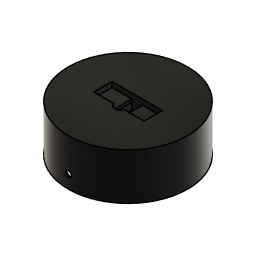
Base V2 - USB C v6 (Autodesk Fusion 360 design; units mm, degrees)
Autodesk Fusion 360 part; units mm, degrees
note: some values were not read from the file. Set by a fixed rule: which face or edge a step refers to.
sketch "Schizzo1" plane through (0, 0, 0) normal (0, 1, 0) x (1, 0, 0)
  circle A0 centre (0, 0) radius 45
  dimension "d1" = 90
  constraint coincident A0.centre origin
  measures "d1" diameter of A0
extrude "Estrusione1" add sketch "Schizzo1" along normal blind 35 makes body 1
shell "Svuotamento1" thickness 4 removed faces 1 at (4.1569, 0, 25.5535) on bodies 1
sketch "Schizzo2" plane through (0, 35, 0) normal (0, 1, 0) x (-1, 0, 0)
  circle A0 centre (0, 0) radius 45
  line L0 (-4, -6.9) -> (4, -6.9)
  line L1 (4, -6.9) -> (4, 6.9)
  line L2 (4, 6.9) -> (-4, 6.9)
  line L3 (-4, 6.9) -> (-4, -6.9)
  line L4 (-4, -6.9) -> (4, 6.9) construction
  line L5 (4, -6.9) -> (-4, 6.9) construction
  dimension "d5" = 8
  dimension "d6" = 13.8
  constraint horizontal L0
  constraint perpendicular L0 L1
  constraint parallel L0 L2
  constraint parallel L1 L3
  constraint coincident L4 A0.centre
  constraint coincident L5 A0.centre
  constraint coincident A0.centre origin
  measures "d5" distance of L1.end L2.end
  measures "d6" distance of L0.end L1.end
extrude "Estrusione2" cut sketch "Schizzo2" against normal blind 40 contours L0 L1 L2 L3 bodies 1
sketch "Schizzo3" plane through (0, 35, 0) normal (0, 1, 0) x (-1, 0, 0)
  line L0 (4, -6.9) -> (-4, -6.9)
  line L1 (-4, -6.9) -> (-4, 6.9)
  line L2 (-4, 6.9) -> (4, 6.9)
  line L3 (4, 6.9) -> (4, -6.9)
  circle A0 centre (0, 0) radius 45
  line L4 (-4, 6.9) -> (-19, 6.9)
  line L5 (-19, 6.9) -> (-19, -6.9)
  line L6 (-19, -6.9) -> (-4, -6.9)
  line L7 (-4, -6.9) -> (-4, 6.9)
  line L8 (4, 6.9) -> (19, 6.9)
  line L9 (19, 6.9) -> (19, -6.9)
  line L10 (19, -6.9) -> (4, -6.9)
  line L11 (4, -6.9) -> (4, 6.9)
  dimension "d9" = 15
  dimension "d10" = 15
  constraint horizontal L4
  constraint vertical L5
  constraint horizontal L6
  constraint vertical L7
  constraint coincident L1.end L2.start
  constraint horizontal L8
  constraint vertical L9
  constraint horizontal L10
  constraint vertical L11
  constraint coincident L2.end L3.start
  measures "d9" distance of L1.end L4.end
  measures "d10" distance of L2.end L8.end
extrude "Estrusione3" add 1 faces at (16.3333, 31, 0) along direction (0, -1, 0) blind 2 on bodies 1 bodies 1
extrude "Estrusione4" cut sketch "Schizzo3" against normal blind 4 contours L3 L8 L9 L10 L11 | L1 L4 L5 L6 L7 bodies 1
sketch "Schizzo4" plane through (0, 35, 0) normal (0, 1, 0) x (-1, 0, 0)
  line L0 (-19, 6.9) -> (19, 6.9)
  line L1 (19, 6.9) -> (19, -6.9)
  line L2 (19, -6.9) -> (-19, -6.9)
  line L3 (-19, -6.9) -> (-19, 6.9)
  circle A0 centre (0, 0) radius 45
  line L4 (-19, 6.9) -> (19, 6.9) construction
  line L5 (0, 6.9) -> (0, 10) construction
  line L6 (0, 6.9) -> (-4, 6.9) construction
  line L7 (0, 6.9) -> (4, 6.9) construction
  arc A1 (4, 6.9) -> (-4, 6.9) centre (0, 5.8694) ccw
  dimension "d15" = 3.1
  constraint coincident L0.start L3.end
  constraint coincident L0.end L1.start
  constraint midpoint L0 L5.start
  constraint perpendicular L4 L5
  constraint coincident L0 L6.end
  constraint perpendicular L5 L6
  constraint coincident L4 L7.end
  constraint coincident L5.end A1
  measures "d15" distance of L5.start L5.end
extrude "Estrusione5" cut sketch "Schizzo4" against normal blind 6 contours L0 A1 bodies 1
ref_plane "Piano di lavoro1" through (0, 14.9575, 45) normal (0, 0, 1) x (-1, 0, 0)
sketch "Schizzo5" plane through (0, 0, 45) normal (0, 0, 1) x (1, 0, 0)
  line L0 (0, 0) -> (0, 32) construction
  circle A0 centre (0, 10) radius 2.25
  dimension "d19" = 4.5
  constraint coincident L0.start origin
  constraint vertical L0
  constraint coincident L0 A0.centre
  measures "d19" diameter of A0
extrude "Estrusione6" cut sketch "Schizzo5" against normal blind 10 bodies 1
ref_plane "Piano di lavoro3" through (0, 14.9017, 45) normal (0, 0, 1) x (-1, 0, 0)
sketch "Schizzo7" plane through (0, 0, 45) normal (0, 0, 1) x (1, 0, 0)
  line L0 (-4.5, 5.5, -6) -> (4.5, 5.5, -6)
  line L1 (4.5, 5.5, -6) -> (4.5, 14.5, -6)
  line L2 (4.5, 14.5, -6) -> (-4.5, 14.5, -6)
  line L3 (-4.5, 14.5, -6) -> (-4.5, 5.5, -6)
  line L4 (-4.5, 5.5, -6) -> (4.5, 14.5, -6) construction
  line L5 (4.5, 5.5, -6) -> (-4.5, 14.5, -6) construction
  point P0 (0, 10)
extrude "Estrusione7" cut sketch "Schizzo7" along normal blind 4 contours L0 L1 L2 L3 in plane through (0, 0, 39) normal (0, 0, 1) bodies 1
fillet "Raccordo1" radius 2 tangency weight 0.1 4 edges at (0, 14.5, 41) (-4.5, 10, 40.7523) (0, 5.5, 41) (4.5, 10, 40.7523) on bodies 1
fillet "Raccordo2" radius 1 tangency weight 0.1 1 edges at (-2.0977, 10.8136, 43) on bodies 1
ref_plane "Piano di lavoro4" through (0, 17.1324, -45) normal (0, 0, -1) x (1, 0, 0)
sketch "Schizzo9" plane through (0, 29, 0) normal (0, -1, 0) x (1, 0, 0)
  circle A0 centre (0, 0) radius 41
  arc A1 (4, 6.9) -> (-4, 6.9) centre (0, 5.8694) ccw
  line L0 (4, 6.9) -> (4, -6.9)
  line L1 (4, -6.9) -> (-4, -6.9)
  line L2 (-4, -6.9) -> (-4, 6.9)
  line L3 (0, 0) -> (25, 0) construction
  line L4 (25, 0) -> (25, -25) construction
  circle A2 centre (25, -25) radius 2
  circle A3 centre (25, -25) radius 3
  dimension "d35" = 25
  dimension "d36" = 25
  dimension "d37" = 4
  dimension "d47" = 1
  constraint coincident A0.centre L3.start
  constraint parallel L1 L3
  constraint perpendicular L3 L4
  constraint coincident L4.end A2.centre
  measures "d35" distance of A0.centre L3.end
  measures "d36" distance of L3.end L4.end
  measures "d37" diameter of A2
extrude "Estrusione9" add sketch "Schizzo9" along normal blind 25 separate body contours A2 makes body 2
sketch "Schizzo10" plane through (0, 29, 0) normal (0, -1, 0) x (1, 0, 0)
  circle A0 centre (0, 0) radius 41
  arc A1 (4, 6.9) -> (-4, 6.9) centre (0, 5.8694) ccw
  line L0 (4, 6.9) -> (4, -6.9)
  line L1 (4, -6.9) -> (-4, -6.9)
  line L2 (-4, -6.9) -> (-4, 6.9)
  line L3 (-6, -8.9) -> (-6, 7.1282)
  arc A2 (6, 7.1282) -> (-6, 7.1282) centre (0, 5.8694) ccw
  line L4 (6, 7.1282) -> (6, -8.9)
  line L5 (6, -8.9) -> (-6, -8.9)
  dimension "d44" = -2
extrude "Estrusione10" add sketch "Schizzo10" along normal blind 5 contours L3 A2 L4 L5 bodies 1
pattern_linear "Serie R3" count 2 spacing 50 along (0, 0, 1) count 2 spacing 50 along (-1, 0, 0) of bodies 2 makes body 3 at (26.9901, 20.6667, 24.8009) makes body 4 at (-23.0099, 20.6667, -25.1991) makes body 5 at (-23.0099, 20.6667, 24.8009)
extrude "Estrusione17" add sketch "Schizzo9" along normal blind 5 separate body contours A3 makes body 6
pattern_linear "Serie R4" count 2 spacing 50 along (-1, 0, 0) count 2 spacing 50 along (0, 0, 1) of bodies 6 makes body 7 at (-22.0037, 25.6667, -25.1495) makes body 8 at (27.9963, 25.6667, 24.8505) makes body 9 at (-22.0037, 25.6667, 24.8505)
ref_plane "Piano di lavoro9" through (-25, 24, -25) normal (0, -1, 0) x (1, 0, 0)
sketch "Schizzo17" plane through (0, 24, 0) normal (0, -1, 0) x (-1, 0, 0)
  circle A0 centre (0, 0) radius 40
  circle A1 centre (-25, 25) radius 2
  circle A2 centre (25, 25) radius 2
  circle A3 centre (25, -25) radius 2
  circle A4 centre (-25, -25) radius 2
  line L0 (-6, 9) -> (6, 9)
  line L1 (6, 9) -> (6, -12)
  line L2 (6, -12) -> (-6, -12)
  line L3 (-6, -12) -> (-6, 9)
  dimension "d88" = 80
  dimension "d89" = 4
  dimension "d90" = 4
  dimension "d91" = 4
  dimension "d92" = 4
  constraint coincident A0.centre origin
  constraint horizontal L0
  constraint vertical L1
  constraint horizontal L2
  constraint vertical L3
  measures "d88" diameter of A0
  measures "d89" diameter of A1
  measures "d90" diameter of A2
  measures "d91" diameter of A3
  measures "d92" diameter of A4
ref_plane "Piano di lavoro10" through (0, 12.3241, -45) normal (0, 0, -1) x (1, 0, 0)
sketch "Schizzo18" plane through (0, 0, -45) normal (0, 0, -1) x (-1, 0, 0)
  line L0 (0, 0) -> (0, 4) construction
  line L1 (0, 4) -> (10.1, 4)
  line L2 (0, 4) -> (-10.1, 4)
  line L3 (-10.1, 4) -> (-10.1, 11.2)
  line L4 (-10.1, 11.2) -> (10, 11.2)
  line L5 (10, 11.2) -> (10.1, 4)
  dimension "d94" = 10.1
  dimension "d95" = 10.1
  dimension "d96" = 7.2
  constraint coincident L0.start origin
  constraint vertical L0
  constraint perpendicular L0 L1
  constraint perpendicular L0 L2
  constraint perpendicular L2 L3
  constraint perpendicular L3 L4
  measures "d94" distance of L0.end L1.end
  measures "d95" distance of L0.end L2.end
  measures "d96" distance of L2.end L3.end
extrude "Estrusione18" add sketch "Schizzo18" against normal blind 8 separate body makes body 10
sketch "Schizzo19" plane through (0, 0, -45) normal (0, 0, -1) x (-1, 0, 0)
  line L0 (-10.1, 4) -> (10.1, 4)
  line L1 (10.1, 4) -> (10, 11.2)
  line L2 (10, 11.2) -> (-10.1, 11.2)
  line L3 (-10.1, 11.2) -> (-10.1, 4)
  line L4 (0, 4) -> (-0.05, 11.2) construction
  line L5 (-10.1, 7.6) -> (10.05, 7.6) construction
  line L6 (-0.025, 7.6) -> (5.9749, 7.6417) construction
  line L7 (-0.025, 7.6) -> (-6.0249, 7.5583) construction
  line L8 (-6.0249, 7.5583) -> (-6.0249, 9.1583) construction
  line L9 (5.9749, 7.6417) -> (5.986, 6.0417) construction
  line L10 (-5.0249, 9.1583) -> (4.986, 9.1583)
  line L11 (5.986, 8.1583) -> (5.986, 7.0417)
  line L12 (4.986, 6.0417) -> (-5.0249, 6.0417)
  line L13 (-6.0249, 7.0417) -> (-6.0249, 8.1583)
  arc A0 (5.986, 8.1583) -> (4.986, 9.1583) centre (4.986, 8.1583) ccw
  arc A1 (-6.0249, 7.0417) -> (-5.0249, 6.0417) centre (-5.0249, 7.0417) ccw
  arc A2 (-5.0249, 9.1583) -> (-6.0249, 8.1583) centre (-5.0249, 8.1583) ccw
  arc A3 (4.986, 6.0417) -> (5.986, 7.0417) centre (4.986, 7.0417) ccw
  dimension "d99" = 6
  dimension "d100" = 6
  dimension "d103" = 1.6
  dimension "d104" = 1.6
  dimension "d105" = 1
  dimension "d106" = 1
  dimension "d107" = 1
  constraint midpoint L0 L4.start
  constraint midpoint L2 L4.end
  constraint midpoint L3 L5.start
  constraint midpoint L1 L5.end
  constraint midpoint L4 L6.start
  constraint perpendicular L4 L6
  constraint perpendicular L4 L7
  constraint perpendicular L5 L8
  constraint perpendicular L6 L9
  constraint horizontal L10
  constraint vertical L11
  constraint horizontal L12
  constraint vertical L13
  constraint tangent L10 A0
  constraint tangent L11 A0
  constraint tangent L12 A1
  constraint tangent L13 A1
  constraint equal A0 A1
  constraint coincident L8.end L10
  constraint coincident L8.end L13
  constraint tangent L10 A2
  constraint tangent L13 A2
  constraint coincident L9.end L11
  constraint coincident L9.end L12
  constraint tangent L11 A3
  constraint tangent L12 A3
  measures "d99" distance of L6.start L6.end
  measures "d100" distance of L6.start L7.end
  measures "d103" distance of L7.end L8.end
  measures "d104" distance of L6.end L9.end
  measures "d105" radius of A0
  measures "d106" radius of A2
  measures "d107" radius of A3
extrude "Estrusione19" cut sketch "Schizzo19" against normal blind 8 contours L10 L11 L12 L13 A0 A1 A2 A3 bodies 1 10
extrude "Estrusione20" cut 1 faces at (8.7416, 7.4139, -37) along direction (0, 0, -1) blind 2 on bodies 10 bodies 10
split "Dividi2" by face at (3.5028, 1.1667, 40.8501) of body 1 bodies 10 makes body 11 at (8.7416, 7.4139, -39)
sketch "Schizzo20" plane through (0, 0, -45) normal (0, 0, -1) x (-1, 0, 0)
  line L0 (4.986, 6.0417) -> (-5.0249, 6.0417)
  arc A0 (-6.0249, 7.0417) -> (-5.0249, 6.0417) centre (-5.0249, 7.0417) ccw
  line L1 (-6.0249, 7.0417) -> (-6.0249, 8.1583)
  arc A1 (-5.0249, 9.1583) -> (-6.0249, 8.1583) centre (-5.0249, 8.1583) ccw
  line L2 (-5.0249, 9.1583) -> (4.986, 9.1583)
  arc A2 (5.986, 8.1583) -> (4.986, 9.1583) centre (4.986, 8.1583) ccw
  line L3 (5.986, 8.1583) -> (5.986, 7.0417)
  arc A3 (4.986, 6.0417) -> (5.986, 7.0417) centre (4.986, 7.0417) ccw
  line L4 (-10.1, 4) -> (10.1, 4)
  line L5 (10.1, 4) -> (10, 11.2)
  line L6 (10, 11.2) -> (-10.1, 11.2)
  line L7 (-10.1, 11.2) -> (-10.1, 4)
  line L8 (0, 0) -> (0, 4) construction
  line L9 (-1.5, -0.356) -> (1.5, -0.356)
  line L10 (1.5, 6.0417) -> (-1.5, 6.0417)
  line L11 (1.5, 6.0417) -> (1.5, -0.356)
  line L12 (-1.5, 6.0417) -> (-1.5, -0.356)
  constraint coincident L8.start origin
  constraint midpoint L4 L8.end
  constraint coincident L0 L10.start
  constraint coincident L0 L10.end
  constraint perpendicular L9 L11
  constraint perpendicular L9 L12
extrude "Estrusione21" cut sketch "Schizzo20" against normal blind 5 contours L0 L4 L10 L11 L12 bodies 1
extrude "Estrusione22" cut sketch "Schizzo20" against normal blind 7 contours L0 L4 L10 L11 L12 | L4 L9 L11 L12 bodies 1 10
hidden bodies 11
